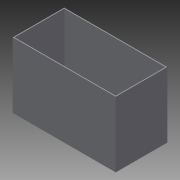
# Autodesk Inventor part: ammoTin
Saved by Autodesk Inventor 2013 (Build 170138000, 138)
## iProperties
Created: 2013-03-14
Part Number: ammoTin
Material: Generic
Document SubType Name: Modeling
Designer: james.eddlestone
Density: 1 g/cm^3
Author: james.eddlestone
Autodesk Inventor part; units mm, degrees
ref_plane "YZ Plane" through (0, 0, 0) normal (1, 0, 0) x (0, 1, 0)
ref_plane "XZ Plane" through (0, 0, 0) normal (0, 1, 0) x (-1, 0, 0)
ref_plane "XY Plane" through (0, 0, 0) normal (0, 0, 1) x (1, 0, 0)
sketch "Sketch1" plane through (0, 0, 0) normal (0, 1, 0) x (-1, 0, 0)
  line L0 (0, 0) -> (279.4, 0)
  line L1 (279.4, 0) -> (279.4, 139.7)
  line L2 (279.4, 139.7) -> (0, 139.7)
  line L3 (0, 139.7) -> (0, 0)
  dimension "d0" = 279.4
  dimension "d1" = 139.7
  constraints: 8 end point, 2 parallel, 1 horizontal, 1 perpendicular
  measures "d0" distance of L2.end L1.end
  measures "d1" distance of L1.end L0.end
extrude "Extrusion1" add sketch "Sketch1" along normal blind 177.8
sketch "Sketch2" plane through (0, 177.8, 0) normal (0, 1, 0) x (1, 0, 0)
  line L0 (0, 0) -> (-279.4, 0) projected
  line L1 (-279.4, 0) -> (-279.4, -139.7) projected
  line L2 (-279.4, -139.7) -> (0, -139.7) projected
  line L3 (0, -139.7) -> (0, 0) projected
  line L4 (-277.0188, -2.3813) -> (-2.3813, -2.3813)
  line L5 (-2.3813, -2.3813) -> (-2.3813, -137.3187)
  line L6 (-2.3813, -137.3187) -> (-277.0188, -137.3187)
  line L7 (-277.0188, -137.3187) -> (-277.0188, -2.3813)
  dimension "d4" = 2.3813
  constraints: 8 end point, 3 other
  measures "d4" distance between parallel lines of L0 L4
extrude "Extrusion2" cut sketch "Sketch2" against normal blind 175.4188 contours L4 L5 L6 L7
body "Solid1"
